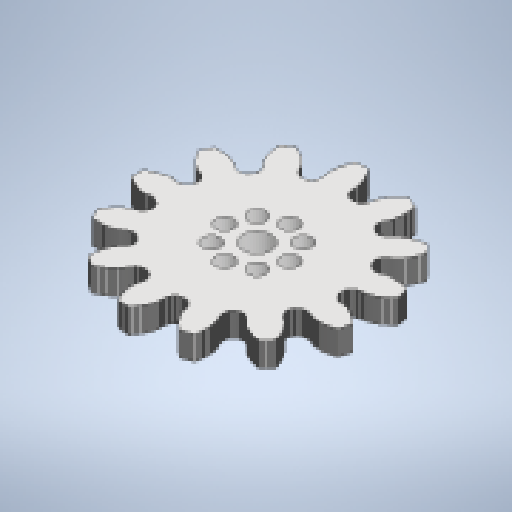
# Autodesk Inventor part: gia1
Saved by Autodesk Inventor 2024 (Build 280153000, 153)
## iProperties
Created: 2024-07-09
Part Number: gia1
Material: 一般
Document SubType Name: Modeling
Designer: right
Density: 1 g/cm^3
Appearance: 既定
Author: right
Autodesk Inventor part; units mm, degrees
(part 1 of 2)
ref_plane "YZ Plane" through (0, 0, 0) normal (1, 0, 0) x (0, 1, 0)
ref_plane "XZ Plane" through (0, 0, 0) normal (0, 1, 0) x (-1, 0, 0)
ref_plane "作業平面1" through (0, 3, 0) normal (0, 1, 0) x (1, 0, 0)
sketch "スケッチ5" plane through (0, 3, 0) normal (0, 1, 0) x (1, 0, 0)
  line L0 (-15.6, 0) -> (15.6, 0)
  line L1 (0, -15.6) -> (0, 15.6)
  line L2 (10.5, 0) -> (10.5, 0.0208)
  line L3 (10.5, 0.0208) -> (10.4999, 0.0416)
  line L4 (10.4999, 0.0416) -> (10.4998, 0.0624)
  line L5 (10.4998, 0.0624) -> (10.4997, 0.0832)
  line L6 (10.4997, 0.0832) -> (10.4995, 0.104)
  line L7 (10.4995, 0.104) -> (10.5112, 0.2583)
  line L8 (10.5112, 0.2583) -> (10.5367, 0.3785)
  line L9 (10.5367, 0.3785) -> (10.5723, 0.481)
  line L10 (10.5723, 0.481) -> (10.6163, 0.5759)
  line L11 (10.6163, 0.5759) -> (10.668, 0.6619)
  line L12 (10.668, 0.6619) -> (10.7267, 0.7429)
  line L13 (10.7267, 0.7429) -> (10.7921, 0.8168)
  line L14 (10.7921, 0.8168) -> (10.8639, 0.8855)
  line L15 (10.8639, 0.8855) -> (10.9417, 0.9492)
  line L16 (10.9417, 0.9492) -> (11.0257, 1.0054)
  line L17 (11.0257, 1.0054) -> (11.1152, 1.0597)
  line L18 (11.1152, 1.0597) -> (11.2106, 1.1065)
  line L19 (11.2106, 1.1065) -> (11.3115, 1.1473)
  line L20 (11.3115, 1.1473) -> (11.4177, 1.1857)
  line L21 (11.4177, 1.1857) -> (11.5292, 1.2172)
  line L22 (11.5292, 1.2172) -> (11.6463, 1.2415)
  line L23 (11.6463, 1.2415) -> (11.7682, 1.263)
  line L24 (11.7682, 1.263) -> (11.895, 1.2797)
  line L25 (11.895, 1.2797) -> (12.027, 1.2893)
  line L26 (12.027, 1.2893) -> (12.1638, 1.2939)
  line L27 (12.1638, 1.2939) -> (12.2934, 1.3227)
  line L28 (12.2934, 1.3227) -> (12.4219, 1.3615)
  line L29 (12.4219, 1.3615) -> (12.5495, 1.4074)
  line L30 (12.5495, 1.4074) -> (12.6764, 1.4593)
  line L31 (12.6764, 1.4593) -> (12.8025, 1.5165)
  line L32 (12.8025, 1.5165) -> (12.928, 1.5786)
  line L33 (12.928, 1.5786) -> (13.0526, 1.6452)
  line L34 (13.0526, 1.6452) -> (13.1766, 1.7162)
  line L35 (13.1766, 1.7162) -> (13.2997, 1.7913)
  line L36 (13.2997, 1.7913) -> (13.422, 1.8703)
  line L37 (13.422, 1.8703) -> (13.5435, 1.9531)
  line L38 (13.5435, 1.9531) -> (13.6642, 2.0397)
  line L39 (13.6642, 2.0397) -> (13.7839, 2.1299)
  line L40 (13.7839, 2.1299) -> (13.9027, 2.2236)
  line L41 (13.9027, 2.2236) -> (14.0206, 2.3209)
  line L42 (14.0206, 2.3209) -> (14.1374, 2.4215)
  line L43 (14.1374, 2.4215) -> (14.2532, 2.5254)
  line L44 (14.2532, 2.5254) -> (14.3679, 2.6326)
  line L45 (14.3679, 2.6326) -> (14.4816, 2.7431)
  line L46 (14.4816, 2.7431) -> (14.594, 2.8567)
  line L47 (14.594, 2.8567) -> (14.5657, 2.9978)
  line L48 (14.5657, 2.9978) -> (14.536, 3.1385)
  line L49 (14.536, 3.1385) -> (14.505, 3.2789)
  line L50 (14.505, 3.2789) -> (14.4726, 3.4191)
  line L51 (14.4726, 3.4191) -> (14.4389, 3.5589)
  line L52 (14.4389, 3.5589) -> (0, 0) construction
  line L53 (0, 0) -> (1.3798, 0.3401) construction
  circle A0 centre (0, 0) radius 13 construction
  line L54 (9.2973, 4.8796) -> (9.3069, 4.8612)
  line L55 (9.3069, 4.8612) -> (9.3165, 4.8427)
  line L56 (9.3165, 4.8427) -> (9.3261, 4.8243)
  line L57 (9.3261, 4.8243) -> (9.3356, 4.8058)
  line L58 (9.3356, 4.8058) -> (9.3451, 4.7873)
  line L59 (9.3451, 4.7873) -> (9.4272, 4.656)
  line L60 (9.4272, 4.656) -> (9.5057, 4.5616)
  line L61 (9.5057, 4.5616) -> (9.5849, 4.4873)
  line L62 (9.5849, 4.4873) -> (9.6679, 4.4237)
  line L63 (9.6679, 4.4237) -> (9.7536, 4.3716)
  line L64 (9.7536, 4.3716) -> (9.8432, 4.3272)
  line L65 (9.8432, 4.3272) -> (9.9355, 4.2921)
  line L66 (9.9355, 4.2921) -> (10.031, 4.2646)
  line L67 (10.031, 4.2646) -> (10.1296, 4.2444)
  line L68 (10.1296, 4.2444) -> (10.23, 4.2337)
  line L69 (10.23, 4.2337) -> (10.3345, 4.2271)
  line L70 (10.3345, 4.2271) -> (10.4407, 4.23)
  line L71 (10.4407, 4.23) -> (10.5491, 4.2408)
  line L72 (10.5491, 4.2408) -> (10.6609, 4.2561)
  line L73 (10.6609, 4.2561) -> (10.7743, 4.2801)
  line L74 (10.7743, 4.2801) -> (10.8892, 4.313)
  line L75 (10.8892, 4.313) -> (11.0071, 4.3506)
  line L76 (11.0071, 4.3506) -> (11.1272, 4.3948)
  line L77 (11.1272, 4.3948) -> (11.2485, 4.4476)
  line L78 (11.2485, 4.4476) -> (11.3718, 4.5071)
  line L79 (11.3718, 4.5071) -> (11.4999, 4.5418)
  line L80 (11.4999, 4.5418) -> (11.6317, 4.5672)
  line L81 (11.6317, 4.5672) -> (11.7661, 4.5858)
  line L82 (11.7661, 4.5858) -> (11.9026, 4.5989)
  line L83 (11.9026, 4.5989) -> (12.0409, 4.6068)
  line L84 (12.0409, 4.6068) -> (12.1808, 4.6101)
  line L85 (12.1808, 4.6101) -> (12.3221, 4.6091)
  line L86 (12.3221, 4.6091) -> (12.4648, 4.6038)
  line L87 (12.4648, 4.6038) -> (12.6087, 4.5946)
  line L88 (12.6087, 4.5946) -> (12.7538, 4.5815)
  line L89 (12.7538, 4.5815) -> (12.8999, 4.5646)
  line L90 (12.8999, 4.5646) -> (13.0469, 4.544)
  line L91 (13.0469, 4.544) -> (13.1949, 4.5198)
  line L92 (13.1949, 4.5198) -> (13.3436, 4.492)
  line L93 (13.3436, 4.492) -> (13.4932, 4.4607)
  line L94 (13.4932, 4.4607) -> (13.6434, 4.4259)
  line L95 (13.6434, 4.4259) -> (13.7942, 4.3877)
  line L96 (13.7942, 4.3877) -> (13.9456, 4.346)
  line L97 (13.9456, 4.346) -> (14.0976, 4.301)
  line L98 (14.0976, 4.301) -> (14.25, 4.2527)
  line L99 (14.25, 4.2527) -> (14.2904, 4.1147)
  line L100 (14.2904, 4.1147) -> (14.3296, 3.9762)
  line L101 (14.3296, 3.9762) -> (14.3673, 3.8375)
  line L102 (14.3673, 3.8375) -> (14.4038, 3.6983)
  line L103 (14.4038, 3.6983) -> (14.4389, 3.5589)
  line L104 (11.0845, 8.0234) -> (11.1511, 8.1561)
  line L105 (9.583, 10.134) -> (9.7277, 10.1785)
  line L106 (9.8746, 10.2203) -> (10.0238, 10.2593)
  line L107 (10.0238, 10.2593) -> (10.1751, 10.2956)
  line L108 (10.1751, 10.2956) -> (10.3285, 10.3291)
  line L109 (9.7277, 10.1785) -> (9.8746, 10.2203)
  line L110 (10.3285, 10.3291) -> (10.484, 10.3598)
  line L111 (10.484, 10.3598) -> (10.6414, 10.3878)
  line L112 (9.4408, 10.0867) -> (9.583, 10.134)
  line L113 (9.301, 10.0366) -> (9.4408, 10.0867)
  line L114 (9.1638, 9.9837) -> (9.301, 10.0366)
  line L115 (8.402, 9.6035) -> (8.5208, 9.6748)
  line L116 (8.5208, 9.6748) -> (8.6431, 9.7428)
  line L117 (8.6431, 9.7428) -> (8.7688, 9.8075)
  line L118 (8.7688, 9.8075) -> (8.8975, 9.8692)
  line L119 (8.8975, 9.8692) -> (9.0293, 9.9279)
  line L120 (9.0293, 9.9279) -> (9.1638, 9.9837)
  line L121 (9.8332, 6.5873) -> (9.9378, 6.661)
  line L122 (9.9378, 6.661) -> (10.0502, 6.7308)
  line L123 (10.0502, 6.7308) -> (10.1692, 6.7985)
  line L124 (10.1692, 6.7985) -> (10.2706, 6.8842)
  line L125 (10.2706, 6.8842) -> (10.3663, 6.9783)
  line L126 (10.3663, 6.9783) -> (10.458, 7.0783)
  line L127 (10.458, 7.0783) -> (10.5462, 7.1832)
  line L128 (10.5462, 7.1832) -> (10.6313, 7.2925)
  line L129 (10.6313, 7.2925) -> (10.7135, 7.4057)
  line L130 (10.7135, 7.4057) -> (10.793, 7.5227)
  line L131 (10.793, 7.5227) -> (10.8697, 7.6431)
  line L132 (9.643, 6.4357) -> (9.7353, 6.5116)
  line L133 (9.7353, 6.5116) -> (9.8332, 6.5873)
  line L134 (9.5588, 6.3559) -> (9.643, 6.4357)
  line L135 (7.8103, 9.0624) -> (7.8932, 9.1656)
  line L136 (7.8932, 9.1656) -> (7.9747, 9.2756)
  line L137 (7.9747, 9.2756) -> (8.072, 9.3659)
  line L138 (8.072, 9.3659) -> (8.1769, 9.4496)
  line L139 (8.1769, 9.4496) -> (8.2872, 9.5285)
  line L140 (8.2872, 9.5285) -> (8.402, 9.6035)
  line L141 (10.8697, 7.6431) -> (10.9439, 7.7667)
  line L142 (10.9439, 7.7667) -> (11.0155, 7.8936)
  line L143 (11.0155, 7.8936) -> (11.0845, 8.0234)
  line L144 (11.1511, 8.1561) -> (11.2152, 8.2916)
  line L145 (11.2152, 8.2916) -> (11.2769, 8.4299)
  line L146 (11.2769, 8.4299) -> (11.336, 8.5707)
  line L147 (11.447, 8.8599) -> (11.4987, 9.0082)
  line L148 (9.4827, 6.2726) -> (9.5588, 6.3559)
  line L149 (7.279, 8.5975) -> (7.3699, 8.6575)
  line L150 (7.3699, 8.6575) -> (7.4618, 8.723)
  line L151 (7.4618, 8.723) -> (7.5511, 8.7969)
  line L152 (7.5511, 8.7969) -> (7.6376, 8.8795)
  line L153 (7.6376, 8.8795) -> (7.7245, 8.9675)
  line L154 (7.7245, 8.9675) -> (7.8103, 9.0624)
  line L155 (9.3496, 6.1039) -> (9.4122, 6.1896)
  line L156 (9.2473, 5.9254) -> (9.2956, 6.0141)
  line L157 (6.7048, 8.4059) -> (6.8028, 8.4177)
  line L158 (6.8028, 8.4177) -> (6.9001, 8.4378)
  line L159 (6.9001, 8.4378) -> (6.9968, 8.4656)
  line L160 (6.9968, 8.4656) -> (7.0907, 8.5029)
  line L161 (7.0907, 8.5029) -> (7.1863, 8.5456)
  line L162 (7.1863, 8.5456) -> (7.279, 8.5975)
  line L163 (5.9818, 8.6295) -> (5.9989, 8.6176)
  line L164 (5.9647, 8.6413) -> (5.9818, 8.6295)
  line L165 (6.0159, 8.6057) -> (6.0329, 8.5938)
  line L166 (5.9989, 8.6176) -> (6.0159, 8.6057)
  line L167 (6.0329, 8.5938) -> (6.0499, 8.5819)
  line L168 (6.6048, 8.4036) -> (6.7048, 8.4059)
  line L169 (6.5047, 8.4099) -> (6.6048, 8.4036)
  line L170 (6.4016, 8.4276) -> (6.5047, 8.4099)
  line L171 (6.297, 8.4566) -> (6.4016, 8.4276)
  line L172 (6.1836, 8.5038) -> (6.297, 8.4566)
  line L173 (6.0499, 8.5819) -> (6.1836, 8.5038)
  line L174 (9.2973, 4.8796) -> (9.2876, 4.898)
  line L175 (9.2485, 4.9714) -> (9.1871, 5.1135)
  line L176 (9.1871, 5.1135) -> (9.1539, 5.2318)
  line L177 (9.1539, 5.2318) -> (9.1378, 5.3391)
  line L178 (9.1378, 5.3391) -> (9.1326, 5.4436)
  line L179 (9.1326, 5.4436) -> (9.1384, 5.5437)
  line L180 (9.1384, 5.5437) -> (9.1528, 5.6427)
  line L181 (9.1528, 5.6427) -> (9.1763, 5.7386)
  line L182 (9.1763, 5.7386) -> (9.208, 5.8328)
  line L183 (9.208, 5.8328) -> (9.2473, 5.9254)
  line L184 (9.2956, 6.0141) -> (9.3496, 6.1039)
  line L185 (9.2583, 4.9531) -> (9.2485, 4.9714)
  line L186 (9.2681, 4.9347) -> (9.2583, 4.9531)
  line L187 (9.2876, 4.898) -> (9.2779, 4.9164)
  line L188 (9.2779, 4.9164) -> (9.2681, 4.9347)
  line L189 (9.4122, 6.1896) -> (9.4827, 6.2726)
  line L190 (11.3927, 8.7141) -> (11.447, 8.8599)
  line L191 (11.4987, 9.0082) -> (11.548, 9.1588)
  line L192 (11.548, 9.1588) -> (11.5948, 9.3117)
  line L193 (11.5948, 9.3117) -> (11.5042, 9.4234)
  line L194 (11.5042, 9.4234) -> (11.4125, 9.5342)
  line L195 (11.4125, 9.5342) -> (11.3198, 9.6442)
  line L196 (11.3198, 9.6442) -> (11.226, 9.7532)
  line L197 (11.226, 9.7532) -> (11.1311, 9.8613)
  line L198 (10.6414, 10.3878) -> (10.7414, 10.2844)
  line L199 (10.7414, 10.2844) -> (10.8403, 10.1801)
  line L200 (10.8403, 10.1801) -> (10.9383, 10.0748)
  line L201 (10.9383, 10.0748) -> (11.0352, 9.9685)
  line L202 (11.0352, 9.9685) -> (11.1311, 9.8613)
  line L203 (11.336, 8.5707) -> (11.3927, 8.7141)
  line L204 (6.0862, 12.2556) -> (6.0835, 12.4041)
  line L205 (3.7758, 13.4267) -> (3.8832, 13.5333)
  line L206 (3.9939, 13.6386) -> (4.1079, 13.7425)
  line L207 (4.1079, 13.7425) -> (4.225, 13.8449)
  line L208 (4.225, 13.8449) -> (4.3453, 13.9459)
  line L209 (3.8832, 13.5333) -> (3.9939, 13.6386)
  line L210 (4.3453, 13.9459) -> (4.4687, 14.0453)
  line L211 (4.4687, 14.0453) -> (4.595, 14.1433)
  line L212 (3.6719, 13.3187) -> (3.7758, 13.4267)
  line L213 (3.5714, 13.2094) -> (3.6719, 13.3187)
  line L214 (3.4745, 13.0987) -> (3.5714, 13.2094)
  line L215 (2.9767, 12.4081) -> (3.0487, 12.5264)
  line L216 (3.0487, 12.5264) -> (3.1254, 12.6434)
  line L217 (3.1254, 12.6434) -> (3.2066, 12.7592)
  line L218 (3.2066, 12.7592) -> (3.2919, 12.8736)
  line L219 (3.2919, 12.8736) -> (3.3813, 12.9868)
  line L220 (3.3813, 12.9868) -> (3.4745, 13.0987)
  line L221 (5.6456, 10.4025) -> (5.704, 10.5164)
  line L222 (5.704, 10.5164) -> (5.7711, 10.6304)
  line L223 (5.7711, 10.6304) -> (5.845, 10.7456)
  line L224 (5.845, 10.7456) -> (5.8949, 10.8686)
  line L225 (5.8949, 10.8686) -> (5.9359, 10.9964)
  line L226 (5.9359, 10.9964) -> (5.9707, 11.1276)
  line L227 (5.9707, 11.1276) -> (6, 11.2615)
  line L228 (6, 11.2615) -> (6.0246, 11.3978)
  line L229 (6.0246, 11.3978) -> (6.0447, 11.5363)
  line L230 (6.0447, 11.5363) -> (6.0607, 11.6767)
  line L231 (6.0607, 11.6767) -> (6.0727, 11.819)
  line L232 (5.5476, 10.1798) -> (5.5941, 10.2899)
  line L233 (5.5941, 10.2899) -> (5.6456, 10.4025)
  line L234 (5.5101, 10.0701) -> (5.5476, 10.1798)
  line L235 (2.7042, 11.654) -> (2.7296, 11.7839)
  line L236 (2.7296, 11.7839) -> (2.7506, 11.9191)
  line L237 (2.7506, 11.9191) -> (2.7948, 12.0443)
  line L238 (2.7948, 12.0443) -> (2.8489, 12.1672)
  line L239 (2.8489, 12.1672) -> (2.9098, 12.2884)
  line L240 (2.9098, 12.2884) -> (2.9767, 12.4081)
  line L241 (6.0727, 11.819) -> (6.0809, 11.963)
  line L242 (6.0809, 11.963) -> (6.0854, 12.1085)
  line L243 (6.0854, 12.1085) -> (6.0862, 12.2556)
  line L244 (6.0835, 12.4041) -> (6.0773, 12.5539)
  line L245 (6.0773, 12.5539) -> (6.0676, 12.7049)
  line L246 (6.0676, 12.7049) -> (6.0546, 12.8571)
  line L247 (6.0184, 13.1648) -> (5.9953, 13.3201)
  line L248 (5.4815, 9.961) -> (5.5101, 10.0701)
  line L249 (2.4497, 10.9955) -> (2.5024, 11.0908)
  line L250 (2.5024, 11.0908) -> (2.5533, 11.1915)
  line L251 (2.5533, 11.1915) -> (2.598, 11.2985)
  line L252 (2.598, 11.2985) -> (2.6362, 11.4117)
  line L253 (2.6362, 11.4117) -> (2.6723, 11.5301)
  line L254 (2.6723, 11.5301) -> (2.7042, 11.654)
  line L255 (5.442, 9.7497) -> (5.4577, 9.8547)
  line L256 (5.4344, 9.5441) -> (5.4359, 9.6451)
  line L257 (2.0304, 10.5589) -> (2.1117, 10.615)
  line L258 (2.1117, 10.615) -> (2.1885, 10.6779)
  line L259 (2.1885, 10.6779) -> (2.2612, 10.7475)
  line L260 (2.2612, 10.7475) -> (2.3271, 10.8242)
  line L261 (2.3271, 10.8242) -> (2.3918, 10.9064)
  line L262 (2.3918, 10.9064) -> (2.4497, 10.9955)
  line L263 (1.2863, 10.4209) -> (1.3069, 10.4183)
  line L264 (1.2656, 10.4234) -> (1.2863, 10.4209)
  line L265 (1.3275, 10.4157) -> (1.3482, 10.4131)
  line L266 (1.3069, 10.4183) -> (1.3275, 10.4157)
  line L267 (1.3482, 10.4131) -> (1.3688, 10.4104)
  line L268 (1.943, 10.5104) -> (2.0304, 10.5589)
  line L269 (1.8514, 10.4695) -> (1.943, 10.5104)
  line L270 (1.7519, 10.4373) -> (1.8514, 10.4695)
  line L271 (1.6458, 10.4143) -> (1.7519, 10.4373)
  line L272 (1.5234, 10.4034) -> (1.6458, 10.4143)
  line L273 (1.3688, 10.4104) -> (1.5234, 10.4034)
  line L274 (5.9647, 8.6413) -> (5.9476, 8.6531)
  line L275 (5.8788, 8.7) -> (5.7584, 8.7973)
  line L276 (5.7584, 8.7973) -> (5.6741, 8.8865)
  line L277 (5.6741, 8.8865) -> (5.6099, 8.9741)
  line L278 (5.6099, 8.9741) -> (5.5568, 9.0642)
  line L279 (5.5568, 9.0642) -> (5.5154, 9.1556)
  line L280 (5.5154, 9.1556) -> (5.4821, 9.2499)
  line L281 (5.4821, 9.2499) -> (5.4584, 9.3457)
  line L282 (5.4584, 9.3457) -> (5.4426, 9.4438)
  line L283 (5.4426, 9.4438) -> (5.4344, 9.5441)
  line L284 (5.4359, 9.6451) -> (5.442, 9.7497)
  line L285 (5.896, 8.6883) -> (5.8788, 8.7)
  line L286 (5.9132, 8.6766) -> (5.896, 8.6883)
  line L287 (5.9476, 8.6531) -> (5.9304, 8.6649)
  line L288 (5.9304, 8.6649) -> (5.9132, 8.6766)
  line L289 (5.4577, 9.8547) -> (5.4815, 9.961)
  line L290 (6.0381, 13.0104) -> (6.0184, 13.1648)
  line L291 (5.9953, 13.3201) -> (5.9689, 13.4764)
  line L292 (5.9689, 13.4764) -> (5.9393, 13.6335)
  line L293 (5.9393, 13.6335) -> (5.8072, 13.6903)
  line L294 (5.8072, 13.6903) -> (5.6745, 13.7458)
  line L295 (5.6745, 13.7458) -> (5.5413, 13.8)
  line L296 (5.5413, 13.8) -> (5.4076, 13.853)
  line L297 (5.4076, 13.853) -> (5.2733, 13.9046)
  line L298 (4.595, 14.1433) -> (4.7316, 14.0982)
  line L299 (4.7316, 14.0982) -> (4.8677, 14.0518)
  line L300 (4.8677, 14.0518) -> (5.0034, 14.004)
  line L301 (5.0034, 14.004) -> (5.1386, 13.955)
  line L302 (5.1386, 13.955) -> (5.2733, 13.9046)
  line L303 (6.0546, 12.8571) -> (6.0381, 13.0104)
  line L304 (-0.3064, 13.6802) -> (-0.3778, 13.8104)
  line L305 (-2.8963, 13.6435) -> (-2.8508, 13.7878)
  line L306 (-2.8017, 13.9324) -> (-2.7491, 14.0774)
  line L307 (-2.7491, 14.0774) -> (-2.693, 14.2225)
  line L308 (-2.693, 14.2225) -> (-2.6334, 14.3678)
  line L309 (-2.8508, 13.7878) -> (-2.8017, 13.9324)
  line L310 (-2.6334, 14.3678) -> (-2.5704, 14.5132)
  line L311 (-2.5704, 14.5132) -> (-2.504, 14.6587)
  line L312 (-2.9382, 13.4995) -> (-2.8963, 13.6435)
  line L313 (-2.9764, 13.356) -> (-2.9382, 13.4995)
  line L314 (-3.0108, 13.213) -> (-2.9764, 13.356)
  line L315 (-3.1306, 12.3701) -> (-3.1219, 12.5084)
  line L316 (-3.1219, 12.5084) -> (-3.1083, 12.6476)
  line L317 (-3.1083, 12.6476) -> (-3.0902, 12.7878)
  line L318 (-3.0902, 12.7878) -> (-3.0678, 12.9289)
  line L319 (-3.0678, 12.9289) -> (-3.0413, 13.0706)
  line L320 (-3.0413, 13.0706) -> (-3.0108, 13.213)
  line L321 (0.1647, 11.8346) -> (0.1634, 11.9625)
  line L322 (0.1634, 11.9625) -> (0.1698, 12.0947)
  line L323 (0.1698, 12.0947) -> (0.1817, 12.2311)
  line L324 (0.1817, 12.2311) -> (0.1688, 12.3632)
  line L325 (0.1688, 12.3632) -> (0.1457, 12.4954)
  line L326 (0.1457, 12.4954) -> (0.1155, 12.6277)
  line L327 (0.1155, 12.6277) -> (0.0793, 12.7599)
  line L328 (0.0793, 12.7599) -> (0.0377, 12.892)
  line L329 (0.0377, 12.892) -> (-0.0088, 13.024)
  line L330 (-0.0088, 13.024) -> (-0.0599, 13.1558)
  line L331 (-0.0599, 13.1558) -> (-0.1154, 13.2873)
  line L332 (0.1814, 11.5919) -> (0.1714, 11.711)
  line L333 (0.1714, 11.711) -> (0.1647, 11.8346)
  line L334 (0.1992, 11.4773) -> (0.1814, 11.5919)
  line L335 (-3.0215, 11.5758) -> (-3.0594, 11.7026)
  line L336 (-3.0594, 11.7026) -> (-3.1035, 11.8322)
  line L337 (-3.1035, 11.8322) -> (-3.1226, 11.9635)
  line L338 (-3.1226, 11.9635) -> (-3.1318, 12.0975)
  line L339 (-3.1318, 12.0975) -> (-3.1342, 12.2331)
  line L340 (-3.1342, 12.2331) -> (-3.1306, 12.3701)
  line L341 (-0.1154, 13.2873) -> (-0.1751, 13.4186)
  line L342 (-0.1751, 13.4186) -> (-0.2388, 13.5496)
  line L343 (-0.2388, 13.5496) -> (-0.3064, 13.6802)
  line L344 (-0.3778, 13.8104) -> (-0.4529, 13.9401)
  line L345 (-0.4529, 13.9401) -> (-0.5316, 14.0694)
  line L346 (-0.5316, 14.0694) -> (-0.6139, 14.1981)
  line L347 (-0.789, 14.4537) -> (-0.8816, 14.5805)
  line L348 (0.2245, 11.3674) -> (0.1992, 11.4773)
  line L349 (-2.9407, 10.8745) -> (-2.9384, 10.9833)
  line L350 (-2.9384, 10.9833) -> (-2.9401, 11.0962)
  line L351 (-2.9401, 11.0962) -> (-2.9502, 11.2117)
  line L352 (-2.9502, 11.2117) -> (-2.969, 11.3297)
  line L353 (-2.969, 11.3297) -> (-2.9921, 11.4513)
  line L354 (-2.9921, 11.4513) -> (-3.0215, 11.5758)
  line L355 (0.2878, 11.1619) -> (0.2528, 11.2622)
  line L356 (0.3766, 10.9764) -> (0.331, 11.0665)
  line L357 (-3.1091, 10.293) -> (-3.0632, 10.3804)
  line L358 (-3.0632, 10.3804) -> (-3.0244, 10.4719)
  line L359 (-3.0244, 10.4719) -> (-2.9924, 10.5673)
  line L360 (-2.9924, 10.5673) -> (-2.9697, 10.6658)
  line L361 (-2.9697, 10.6658) -> (-2.9506, 10.7687)
  line L362 (-2.9506, 10.7687) -> (-2.9407, 10.8745)
  line L363 (-3.7039, 9.825) -> (-3.6844, 9.8323)
  line L364 (-3.7234, 9.8177) -> (-3.7039, 9.825)
  line L365 (-3.665, 9.8396) -> (-3.6455, 9.8469)
  line L366 (-3.6844, 9.8323) -> (-3.665, 9.8396)
  line L367 (-3.6455, 9.8469) -> (-3.626, 9.8541)
  line L368 (-3.164, 10.2095) -> (-3.1091, 10.293)
  line L369 (-3.2261, 10.1307) -> (-3.164, 10.2095)
  line L370 (-3.2992, 10.0559) -> (-3.2261, 10.1307)
  line L371 (-3.3825, 9.9862) -> (-3.2992, 10.0559)
  line L372 (-3.4858, 9.9197) -> (-3.3825, 9.9862)
  line L373 (-3.626, 9.8541) -> (-3.4858, 9.9197)
  line L374 (1.2656, 10.4234) -> (1.245, 10.4259)
  line L375 (1.1624, 10.4355) -> (1.0105, 10.4657)
  line L376 (1.0105, 10.4657) -> (0.8944, 10.5055)
  line L377 (0.8944, 10.5055) -> (0.7968, 10.5532)
  line L378 (0.7968, 10.5532) -> (0.7079, 10.6083)
  line L379 (0.7079, 10.6083) -> (0.6288, 10.67)
  line L380 (0.6288, 10.67) -> (0.5555, 10.738)
  line L381 (0.5555, 10.738) -> (0.49, 10.8119)
  line L382 (0.49, 10.8119) -> (0.4304, 10.8914)
  line L383 (0.4304, 10.8914) -> (0.3766, 10.9764)
  line L384 (0.331, 11.0665) -> (0.2878, 11.1619)
  line L385 (1.183, 10.4331) -> (1.1624, 10.4355)
  line L386 (1.2037, 10.4308) -> (1.183, 10.4331)
  line L387 (1.245, 10.4259) -> (1.2243, 10.4284)
  line L388 (1.2243, 10.4284) -> (1.2037, 10.4308)
  line L389 (0.2528, 11.2622) -> (0.2245, 11.3674)
  line L390 (-0.6997, 14.3262) -> (-0.789, 14.4537)
  line L391 (-0.8816, 14.5805) -> (-0.9775, 14.7066)
  line L392 (-0.9775, 14.7066) -> (-1.0768, 14.832)
  line L393 (-1.0768, 14.832) -> (-1.2202, 14.8209)
  line L394 (-1.2202, 14.8209) -> (-1.3635, 14.8084)
  line L395 (-1.3635, 14.8084) -> (-1.5066, 14.7945)
  line L396 (-1.5066, 14.7945) -> (-1.6496, 14.7792)
  line L397 (-1.6496, 14.7792) -> (-1.7925, 14.7626)
  line L398 (-2.504, 14.6587) -> (-2.3621, 14.6822)
  line L399 (-2.3621, 14.6822) -> (-2.22, 14.7044)
  line L400 (-2.22, 14.7044) -> (-2.0777, 14.7251)
  line L401 (-2.0777, 14.7251) -> (-1.9352, 14.7446)
  line L402 (-1.9352, 14.7446) -> (-1.7925, 14.7626)
  line L403 (-0.6139, 14.1981) -> (-0.6997, 14.3262)
  line L404 (-6.6288, 11.9708) -> (-6.7525, 12.0529)
  line L405 (-8.905, 10.7347) -> (-8.9318, 10.8836)
  line L406 (-8.9555, 11.0345) -> (-8.9763, 11.1873)
  line L407 (-8.9763, 11.1873) -> (-8.994, 11.3419)
  line L408 (-8.994, 11.3419) -> (-9.0088, 11.4983)
  line L409 (-8.9318, 10.8836) -> (-8.9555, 11.0345)
  line L410 (-9.0088, 11.4983) -> (-9.0206, 11.6563)
  line L411 (-9.0206, 11.6563) -> (-9.0294, 11.8159)
  line L412 (-8.8752, 10.5878) -> (-8.905, 10.7347)
  line L413 (-8.8423, 10.443) -> (-8.8752, 10.5878)
  line L414 (-8.8063, 10.3004) -> (-8.8423, 10.443)
  line L415 (-8.5207, 9.4983) -> (-8.5772, 9.6248)
  line L416 (-8.5772, 9.6248) -> (-8.6299, 9.7544)
  line L417 (-8.6299, 9.7544) -> (-8.679, 9.887)
  line L418 (-8.679, 9.887) -> (-8.7247, 10.0223)
  line L419 (-8.7247, 10.0223) -> (-8.7671, 10.1601)
  line L420 (-8.7671, 10.1601) -> (-8.8063, 10.3004)
  line L421 (-5.354, 10.5555) -> (-5.4146, 10.6682)
  line L422 (-5.4146, 10.6682) -> (-5.4703, 10.7883)
  line L423 (-5.4703, 10.7883) -> (-5.5231, 10.9145)
  line L424 (-5.5231, 10.9145) -> (-5.596, 11.0255)
  line L425 (-5.596, 11.0255) -> (-5.6779, 11.1319)
  line L426 (-5.6779, 11.1319) -> (-5.7661, 11.2349)
  line L427 (-5.7661, 11.2349) -> (-5.8596, 11.3352)
  line L428 (-5.8596, 11.3352) -> (-5.9578, 11.4328)
  line L429 (-5.9578, 11.4328) -> (-6.0603, 11.5281)
  line L430 (-6.0603, 11.5281) -> (-6.1669, 11.621)
  line L431 (-6.1669, 11.621) -> (-6.2771, 11.7117)
  line L432 (-5.2264, 10.3484) -> (-5.2906, 10.4492)
  line L433 (-5.2906, 10.4492) -> (-5.354, 10.5555)
  line L434 (-5.1574, 10.2552) -> (-5.2264, 10.3484)
  line L435 (-8.0549, 8.8457) -> (-8.1474, 8.9404)
  line L436 (-8.1474, 8.9404) -> (-8.2467, 9.0346)
  line L437 (-8.2467, 9.0346) -> (-8.3246, 9.1421)
  line L438 (-8.3246, 9.1421) -> (-8.3951, 9.2563)
  line L439 (-8.3951, 9.2563) -> (-8.4602, 9.3753)
  line L440 (-8.4602, 9.3753) -> (-8.5207, 9.4983)
  line L441 (-6.2771, 11.7117) -> (-6.391, 11.8002)
  line L442 (-6.391, 11.8002) -> (-6.5083, 11.8866)
  line L443 (-6.5083, 11.8866) -> (-6.6288, 11.9708)
  line L444 (-6.7525, 12.0529) -> (-6.8793, 12.1329)
  line L445 (-6.8793, 12.1329) -> (-7.0091, 12.2108)
  line L446 (-7.0091, 12.2108) -> (-7.1418, 12.2865)
  line L447 (-7.4156, 12.4315) -> (-7.5565, 12.5007)
  line L448 (-5.0839, 10.1696) -> (-5.1574, 10.2552)
  line L449 (-7.6575, 8.2622) -> (-7.706, 8.3597)
  line L450 (-7.706, 8.3597) -> (-7.76, 8.4588)
  line L451 (-7.76, 8.4588) -> (-7.8226, 8.5564)
  line L452 (-7.8226, 8.5564) -> (-7.8941, 8.6522)
  line L453 (-7.8941, 8.6522) -> (-7.9711, 8.7491)
  line L454 (-7.9711, 8.7491) -> (-8.0549, 8.8457)
  line L455 (-4.9324, 10.0171) -> (-5.0099, 10.0897)
  line L456 (-4.7676, 9.8941) -> (-4.8498, 9.9527)
  line L457 (-7.5364, 7.6692) -> (-7.5364, 7.7679)
  line L458 (-7.5364, 7.7679) -> (-7.5445, 7.8669)
  line L459 (-7.5445, 7.8669) -> (-7.5605, 7.9662)
  line L460 (-7.5605, 7.9662) -> (-7.5862, 8.064)
  line L461 (-7.5862, 8.064) -> (-7.6171, 8.164)
  line L462 (-7.6171, 8.164) -> (-7.6575, 8.2622)
  line L463 (-7.8456, 6.9783) -> (-7.8317, 6.9939)
  line L464 (-7.8594, 6.9628) -> (-7.8456, 6.9783)
  line L465 (-7.8179, 7.0094) -> (-7.804, 7.0248)
  line L466 (-7.8317, 6.9939) -> (-7.8179, 7.0094)
  line L467 (-7.804, 7.0248) -> (-7.79, 7.0403)
  line L468 (-7.5462, 7.5696) -> (-7.5364, 7.6692)
  line L469 (-7.5645, 7.471) -> (-7.5462, 7.5696)
  line L470 (-7.5945, 7.3708) -> (-7.5645, 7.471)
  line L471 (-7.6359, 7.2704) -> (-7.5945, 7.3708)
  line L472 (-7.6964, 7.1636) -> (-7.6359, 7.2704)
  line L473 (-7.79, 7.0403) -> (-7.6964, 7.1636)
  line L474 (-3.7234, 9.8177) -> (-3.7428, 9.8103)
  line L475 (-3.8204, 9.7803) -> (-3.9689, 9.7365)
  line L476 (-3.9689, 9.7365) -> (-4.0902, 9.7178)
  line L477 (-4.0902, 9.7178) -> (-4.1988, 9.7147)
  line L478 (-4.1988, 9.7147) -> (-4.3031, 9.7222)
  line L479 (-4.3031, 9.7222) -> (-4.4018, 9.74)
  line L480 (-4.4018, 9.74) -> (-4.4983, 9.7662)
  line L481 (-4.4983, 9.7662) -> (-4.5907, 9.8011)
  line L482 (-4.5907, 9.8011) -> (-4.6803, 9.8439)
  line L483 (-4.6803, 9.8439) -> (-4.7676, 9.8941)
  line L484 (-4.8498, 9.9527) -> (-4.9324, 10.0171)
  line L485 (-3.801, 9.7879) -> (-3.8204, 9.7803)
  line L486 (-3.7816, 9.7954) -> (-3.801, 9.7879)
  line L487 (-3.7428, 9.8103) -> (-3.7622, 9.8028)
  line L488 (-3.7622, 9.8028) -> (-3.7816, 9.7954)
  line L489 (-5.0099, 10.0897) -> (-5.0839, 10.1696)
  line L490 (-7.2773, 12.36) -> (-7.4156, 12.4315)
  line L491 (-7.5565, 12.5007) -> (-7.7001, 12.5678)
  line L492 (-7.7001, 12.5678) -> (-7.8462, 12.6326)
  line L493 (-7.8462, 12.6326) -> (-7.968, 12.5562)
  line L494 (-7.968, 12.5562) -> (-8.0891, 12.4785)
  line L495 (-8.0891, 12.4785) -> (-8.2094, 12.3997)
  line L496 (-8.2094, 12.3997) -> (-8.3289, 12.3197)
  line L497 (-8.3289, 12.3197) -> (-8.4477, 12.2386)
  line L498 (-9.0294, 11.8159) -> (-8.9147, 11.9027)
  line L499 (-8.9147, 11.9027) -> (-8.7992, 11.9884)
  line L500 (-8.7992, 11.9884) -> (-8.6828, 12.0729)
  line L501 (-8.6828, 12.0729) -> (-8.5657, 12.1563)
  line L502 (-8.5657, 12.1563) -> (-8.4477, 12.2386)
  line L503 (-7.1418, 12.2865) -> (-7.2773, 12.36)
  line L504 (-11.4326, 7.5191) -> (-11.5804, 7.5343)
  line L505 (-12.8737, 5.3667) -> (-12.9666, 5.4862)
  line L506 (-13.0577, 5.6088) -> (-13.1471, 5.7344)
  line L507 (-13.1471, 5.7344) -> (-13.2347, 5.863)
  line L508 (-13.2347, 5.863) -> (-13.3204, 5.9946)
  line L509 (-12.9666, 5.4862) -> (-13.0577, 5.6088)
  line L510 (-13.3204, 5.9946) -> (-13.4043, 6.1291)
  line L511 (-13.4043, 6.1291) -> (-13.4863, 6.2663)
  line L512 (-12.779, 5.2505) -> (-12.8737, 5.3667)
  line L513 (-12.6826, 5.1376) -> (-12.779, 5.2505)
  line L514 (-12.5844, 5.028) -> (-12.6826, 5.1376)
  line L515 (-11.9588, 4.4506) -> (-12.0676, 4.5363)
  line L516 (-12.0676, 4.5363) -> (-12.1745, 4.6266)
  line L517 (-12.1745, 4.6266) -> (-12.2796, 4.7211)
  line L518 (-12.2796, 4.7211) -> (-12.383, 4.8197)
  line L519 (-12.383, 4.8197) -> (-12.4846, 4.922)
  line L520 (-12.4846, 4.922) -> (-12.5844, 5.028)
  line L521 (-9.6461, 6.8583) -> (-9.7521, 6.93)
  line L522 (-9.7521, 6.93) -> (-9.8573, 7.0104)
  line L523 (-9.8573, 7.0104) -> (-9.9627, 7.0976)
  line L524 (-9.9627, 7.0976) -> (-10.0788, 7.162)
  line L525 (-10.0788, 7.162) -> (-10.2007, 7.2181)
  line L526 (-10.2007, 7.2181) -> (-10.3267, 7.2684)
  line L527 (-10.3267, 7.2684) -> (-10.4561, 7.3137)
  line L528 (-10.4561, 7.3137) -> (-10.5885, 7.3545)
  line L529 (-10.5885, 7.3545) -> (-10.7235, 7.3912)
  line L530 (-10.7235, 7.3912) -> (-10.861, 7.424)
  line L531 (-10.861, 7.424) -> (-11.0008, 7.4531)
  line L532 (-9.4369, 6.7342) -> (-9.5406, 6.7936)
  line L533 (-9.5406, 6.7936) -> (-9.6461, 6.8583)
  line L534 (-9.3325, 6.6838) -> (-9.4369, 6.7342)
  line L535 (-11.2431, 4.0892) -> (-11.369, 4.13)
  line L536 (-11.369, 4.13) -> (-11.5007, 4.1673)
  line L537 (-11.5007, 4.1673) -> (-11.6196, 4.2262)
  line L538 (-11.6196, 4.2262) -> (-11.7351, 4.2947)
  line L539 (-11.7351, 4.2947) -> (-11.848, 4.3698)
  line L540 (-11.848, 4.3698) -> (-11.9588, 4.4506)
  line L541 (-11.0008, 7.4531) -> (-11.1428, 7.4786)
  line L542 (-11.1428, 7.4786) -> (-11.2868, 7.5005)
  line L543 (-11.2868, 7.5005) -> (-11.4326, 7.5191)
  line L544 (-11.5804, 7.5343) -> (-11.7298, 7.5462)
  line L545 (-11.7298, 7.5462) -> (-11.8809, 7.5548)
  line L546 (-11.8809, 7.5548) -> (-12.0336, 7.5602)
  line L547 (-12.3433, 7.5613) -> (-12.5003, 7.5572)
  line L548 (-9.2276, 6.6422) -> (-9.3325, 6.6838)
  line L549 (-10.62, 3.7572) -> (-10.7083, 3.821)
  line L550 (-10.7083, 3.821) -> (-10.8021, 3.8837)
  line L551 (-10.8021, 3.8837) -> (-10.9029, 3.9409)
  line L552 (-10.9029, 3.9409) -> (-11.0107, 3.9925)
  line L553 (-11.0107, 3.9925) -> (-11.1239, 4.0426)
  line L554 (-11.1239, 4.0426) -> (-11.2431, 4.0892)
  line L555 (-9.0226, 6.5775) -> (-9.125, 6.6057)
  line L556 (-8.8195, 6.5452) -> (-8.9196, 6.5589)
  line L557 (-10.2372, 3.2883) -> (-10.283, 3.3758)
  line L558 (-10.283, 3.3758) -> (-10.3363, 3.4597)
  line L559 (-10.3363, 3.4597) -> (-10.3966, 3.5402)
  line L560 (-10.3966, 3.5402) -> (-10.4647, 3.6148)
  line L561 (-10.4647, 3.6148) -> (-10.5386, 3.689)
  line L562 (-10.5386, 3.689) -> (-10.62, 3.7572)
  line L563 (-10.1899, 2.533) -> (-10.1849, 2.5532)
  line L564 (-10.1949, 2.5128) -> (-10.1899, 2.533)
  line L565 (-10.1798, 2.5733) -> (-10.1747, 2.5935)
  line L566 (-10.1849, 2.5532) -> (-10.1798, 2.5733)
  line L567 (-10.1747, 2.5935) -> (-10.1695, 2.6136)
  line L568 (-10.1996, 3.1957) -> (-10.2372, 3.2883)
  line L569 (-10.17, 3.0999) -> (-10.1996, 3.1957)
  line L570 (-10.15, 2.9972) -> (-10.17, 3.0999)
  line L571 (-10.14, 2.8891) -> (-10.15, 2.9972)
  line L572 (-10.1439, 2.7663) -> (-10.14, 2.8891)
  line L573 (-10.1695, 2.6136) -> (-10.1439, 2.7663)
  line L574 (-7.8594, 6.9628) -> (-7.8731, 6.9472)
  line L575 (-7.9279, 6.8846) -> (-8.039, 6.7768)
  line L576 (-8.039, 6.7768) -> (-8.1378, 6.7039)
  line L577 (-8.1378, 6.7039) -> (-8.2325, 6.6507)
  line L578 (-8.2325, 6.6507) -> (-8.3283, 6.6088)
  line L579 (-8.3283, 6.6088) -> (-8.424, 6.5788)
  line L580 (-8.424, 6.5788) -> (-8.5217, 6.5571)
  line L581 (-8.5217, 6.5571) -> (-8.6196, 6.5451)
  line L582 (-8.6196, 6.5451) -> (-8.7189, 6.5413)
  line L583 (-8.7189, 6.5413) -> (-8.8195, 6.5452)
  line L584 (-8.9196, 6.5589) -> (-9.0226, 6.5775)
  line L585 (-7.9143, 6.9003) -> (-7.9279, 6.8846)
  line L586 (-7.9006, 6.916) -> (-7.9143, 6.9003)
  line L587 (-7.8731, 6.9472) -> (-7.8869, 6.9316)
  line L588 (-7.8869, 6.9316) -> (-7.9006, 6.916)
  line L589 (-9.125, 6.6057) -> (-9.2276, 6.6422)
  line L590 (-12.1877, 7.5623) -> (-12.3433, 7.5613)
  line L591 (-12.5003, 7.5572) -> (-12.6586, 7.5498)
  line L592 (-12.6586, 7.5498) -> (-12.8182, 7.5393)
  line L593 (-12.8182, 7.5393) -> (-12.8905, 7.415)
  line L594 (-12.8905, 7.415) -> (-12.9616, 7.29)
  line L595 (-12.9616, 7.29) -> (-13.0315, 7.1643)
  line L596 (-13.0315, 7.1643) -> (-13.1002, 7.0379)
  line L597 (-13.1002, 7.0379) -> (-13.1676, 6.9109)
  line L598 (-13.4863, 6.2663) -> (-13.4251, 6.3964)
  line L599 (-13.4251, 6.3964) -> (-13.3626, 6.526)
  line L600 (-13.3626, 6.526) -> (-13.2988, 6.6549)
  line L601 (-13.2988, 6.6549) -> (-13.2338, 6.7832)
  line L602 (-13.2338, 6.7832) -> (-13.1676, 6.9109)
  line L603 (-12.0336, 7.5602) -> (-12.1877, 7.5623)
  line L604 (-13.6174, 1.3448) -> (-13.7552, 1.2896)
  line L605 (-13.8931, -1.2307) -> (-14.0309, -1.1681)
  line L606 (-14.1686, -1.1019) -> (-14.3061, -1.0322)
  line L607 (-14.3061, -1.0322) -> (-14.4434, -0.959)
  line L608 (-14.4434, -0.959) -> (-14.5805, -0.8823)
  line L609 (-14.0309, -1.1681) -> (-14.1686, -1.1019)
  line L610 (-14.5805, -0.8823) -> (-14.7172, -0.8023)
  line L611 (-14.7172, -0.8023) -> (-14.8536, -0.7189)
  line L612 (-13.7552, -1.2896) -> (-13.8931, -1.2307)
  line L613 (-13.6174, -1.3448) -> (-13.7552, -1.2896)
  line L614 (-13.4796, -1.3962) -> (-13.6174, -1.3448)
  line L615 (-12.6573, -1.6167) -> (-12.7935, -1.5914)
  line L616 (-12.7935, -1.5914) -> (-12.9301, -1.5611)
  line L617 (-12.9301, -1.5611) -> (-13.0671, -1.5263)
  line L618 (-13.0671, -1.5263) -> (-13.2044, -1.487)
  line L619 (-13.2044, -1.487) -> (-13.3419, -1.4436)
  line L620 (-13.3419, -1.4436) -> (-13.4796, -1.3962)
  line L621 (-11.7285, 1.59) -> (-11.8556, 1.6041)
  line L622 (-11.8556, 1.6041) -> (-11.9861, 1.6265)
  line L623 (-11.9861, 1.6265) -> (-12.12, 1.6547)
  line L624 (-12.12, 1.6547) -> (-12.2527, 1.6578)
  line L625 (-12.2527, 1.6578) -> (-12.3867, 1.6508)
  line L626 (-12.3867, 1.6508) -> (-12.5217, 1.6368)
  line L627 (-12.5217, 1.6368) -> (-12.6573, 1.6167)
  line L628 (-12.6573, 1.6167) -> (-12.7935, 1.5914)
  line L629 (-12.7935, 1.5914) -> (-12.9301, 1.5611)
  line L630 (-12.9301, 1.5611) -> (-13.0671, 1.5263)
  line L631 (-13.0671, 1.5263) -> (-13.2044, 1.487)
  line L632 (-11.4855, 1.5773) -> (-11.605, 1.5817)
  line L633 (-11.605, 1.5817) -> (-11.7285, 1.59)
  line L634 (-11.3696, 1.5812) -> (-11.4855, 1.5773)
  line L635 (-11.8556, -1.6041) -> (-11.9861, -1.6265)
  line L636 (-11.9861, -1.6265) -> (-12.12, -1.6547)
  line L637 (-12.12, -1.6547) -> (-12.2527, -1.6578)
  line L638 (-12.2527, -1.6578) -> (-12.3867, -1.6508)
  line L639 (-12.3867, -1.6508) -> (-12.5217, -1.6368)
  line L640 (-12.5217, -1.6368) -> (-12.6573, -1.6167)
  line L641 (-13.2044, 1.487) -> (-13.3419, 1.4436)
  line L642 (-13.3419, 1.4436) -> (-13.4796, 1.3962)
  line L643 (-13.4796, 1.3962) -> (-13.6174, 1.3448)
  line L644 (-13.7552, 1.2896) -> (-13.8931, 1.2307)
  line L645 (-13.8931, 1.2307) -> (-14.0309, 1.1681)
  line L646 (-14.0309, 1.1681) -> (-14.1686, 1.1019)
  line L647 (-14.4434, 0.959) -> (-14.5805, 0.8823)
  line L648 (-11.2574, 1.5931) -> (-11.3696, 1.5812)
  line L649 (-11.1496, -1.6085) -> (-11.2574, -1.5931)
  line L650 (-11.2574, -1.5931) -> (-11.3696, -1.5812)
  line L651 (-11.3696, -1.5812) -> (-11.4855, -1.5773)
  line L652 (-11.4855, -1.5773) -> (-11.605, -1.5817)
  line L653 (-11.605, -1.5817) -> (-11.7285, -1.59)
  line L654 (-11.7285, -1.59) -> (-11.8556, -1.6041)
  line L655 (-11.0458, 1.6311) -> (-11.1496, 1.6085)
  line L656 (-10.8509, 1.6969) -> (-10.946, 1.6625)
  line L657 (-10.5928, -1.8458) -> (-10.674, -1.7896)
  line L658 (-10.674, -1.7896) -> (-10.7601, -1.7401)
  line L659 (-10.7601, -1.7401) -> (-10.8509, -1.6969)
  line L660 (-10.8509, -1.6969) -> (-10.946, -1.6625)
  line L661 (-10.946, -1.6625) -> (-11.0458, -1.6311)
  line L662 (-11.0458, -1.6311) -> (-11.1496, -1.6085)
  line L663 (-10.1998, -2.4926) -> (-10.2048, -2.4724)
  line L664 (-10.1949, -2.5128) -> (-10.1998, -2.4926)
  line L665 (-10.2096, -2.4522) -> (-10.2145, -2.432)
  line L666 (-10.2048, -2.4724) -> (-10.2096, -2.4522)
  line L667 (-10.2145, -2.432) -> (-10.2193, -2.4118)
  line L668 (-10.5164, -1.9104) -> (-10.5928, -1.8458)
  line L669 (-10.4456, -1.9814) -> (-10.5164, -1.9104)
  line L670 (-10.3802, -2.0631) -> (-10.4456, -1.9814)
  line L671 (-10.3211, -2.1541) -> (-10.3802, -2.0631)
  line L672 (-10.2676, -2.2647) -> (-10.3211, -2.1541)
  line L673 (-10.2193, -2.4118) -> (-10.2676, -2.2647)
  line L674 (-10.1949, 2.5128) -> (-10.1998, 2.4926)
  line L675 (-10.2193, 2.4118) -> (-10.2676, 2.2647)
  line L676 (-10.2676, 2.2647) -> (-10.3211, 2.1541)
  line L677 (-10.3211, 2.1541) -> (-10.3802, 2.0631)
  line L678 (-10.3802, 2.0631) -> (-10.4456, 1.9814)
  line L679 (-10.4456, 1.9814) -> (-10.5164, 1.9104)
  line L680 (-10.5164, 1.9104) -> (-10.5928, 1.8458)
  line L681 (-10.5928, 1.8458) -> (-10.674, 1.7896)
  line L682 (-10.674, 1.7896) -> (-10.7601, 1.7401)
  line L683 (-10.7601, 1.7401) -> (-10.8509, 1.6969)
  line L684 (-10.946, 1.6625) -> (-11.0458, 1.6311)
  line L685 (-10.2145, 2.432) -> (-10.2193, 2.4118)
  line L686 (-10.2096, 2.4522) -> (-10.2145, 2.432)
  line L687 (-10.1998, 2.4926) -> (-10.2048, 2.4724)
  line L688 (-10.2048, 2.4724) -> (-10.2096, 2.4522)
  line L689 (-11.1496, 1.6085) -> (-11.2574, 1.5931)
  line L690 (-14.3061, 1.0322) -> (-14.4434, 0.959)
  line L691 (-14.5805, 0.8823) -> (-14.7172, 0.8023)
  line L692 (-14.7172, 0.8023) -> (-14.8536, 0.7189)
  line L693 (-14.8536, 0.7189) -> (-14.8599, 0.5752)
  line L694 (-14.8599, 0.5752) -> (-14.8647, 0.4314)
  line L695 (-14.8647, 0.4314) -> (-14.8682, 0.2876)
  line L696 (-14.8682, 0.2876) -> (-14.8703, 0.1438)
  line L697 (-14.8703, 0.1438) -> (-14.871, 0)
  line L698 (-14.8536, -0.7189) -> (-14.8599, -0.5752)
  line L699 (-14.8599, -0.5752) -> (-14.8647, -0.4314)
  line L700 (-14.8647, -0.4314) -> (-14.8682, -0.2876)
  line L701 (-14.8682, -0.2876) -> (-14.8703, -0.1438)
  line L702 (-14.8703, -0.1438) -> (-14.871, 0)
  line L703 (-14.1686, 1.1019) -> (-14.3061, 1.0322)
  line L704 (-12.6826, -5.1376) -> (-12.779, -5.2505)
  line L705 (-11.7298, -7.5462) -> (-11.8809, -7.5548)
  line L706 (-12.0336, -7.5602) -> (-12.1877, -7.5623)
  line L707 (-12.1877, -7.5623) -> (-12.3433, -7.5613)
  line L708 (-12.3433, -7.5613) -> (-12.5003, -7.5572)
  line L709 (-11.8809, -7.5548) -> (-12.0336, -7.5602)
  line L710 (-12.5003, -7.5572) -> (-12.6586, -7.5498)
  line L711 (-12.6586, -7.5498) -> (-12.8182, -7.5393)
  line L712 (-11.5804, -7.5343) -> (-11.7298, -7.5462)
  line L713 (-11.4326, -7.5191) -> (-11.5804, -7.5343)
  line L714 (-11.2868, -7.5005) -> (-11.4326, -7.5191)
  line L715 (-10.4561, -7.3137) -> (-10.5885, -7.3545)
  line L716 (-10.5885, -7.3545) -> (-10.7235, -7.3912)
  line L717 (-10.7235, -7.3912) -> (-10.861, -7.424)
  line L718 (-10.861, -7.424) -> (-11.0008, -7.4531)
  line L719 (-11.0008, -7.4531) -> (-11.1428, -7.4786)
  line L720 (-11.1428, -7.4786) -> (-11.2868, -7.5005)
  line L721 (-11.1239, -4.0426) -> (-11.2431, -4.0892)
  line L722 (-11.2431, -4.0892) -> (-11.369, -4.13)
  line L723 (-11.369, -4.13) -> (-11.5007, -4.1673)
  line L724 (-11.5007, -4.1673) -> (-11.6196, -4.2262)
  line L725 (-11.6196, -4.2262) -> (-11.7351, -4.2947)
  line L726 (-11.7351, -4.2947) -> (-11.848, -4.3698)
  line L727 (-11.848, -4.3698) -> (-11.9588, -4.4506)
  line L728 (-11.9588, -4.4506) -> (-12.0676, -4.5363)
  line L729 (-12.0676, -4.5363) -> (-12.1745, -4.6266)
  line L730 (-12.1745, -4.6266) -> (-12.2796, -4.7211)
  line L731 (-12.2796, -4.7211) -> (-12.383, -4.8197)
  line L732 (-10.9029, -3.9409) -> (-11.0107, -3.9925)
  line L733 (-11.0107, -3.9925) -> (-11.1239, -4.0426)
  line L734 (-10.8021, -3.8837) -> (-10.9029, -3.9409)
  line L735 (-9.7521, -6.93) -> (-9.8573, -7.0104)
  line L736 (-9.8573, -7.0104) -> (-9.9627, -7.0976)
  line L737 (-9.9627, -7.0976) -> (-10.0788, -7.162)
  line L738 (-10.0788, -7.162) -> (-10.2007, -7.2181)
  line L739 (-10.2007, -7.2181) -> (-10.3267, -7.2684)
  line L740 (-10.3267, -7.2684) -> (-10.4561, -7.3137)
  line L741 (-12.383, -4.8197) -> (-12.4846, -4.922)
  line L742 (-12.4846, -4.922) -> (-12.5844, -5.028)
  line L743 (-12.5844, -5.028) -> (-12.6826, -5.1376)
  line L744 (-12.779, -5.2505) -> (-12.8737, -5.3667)
  line L745 (-12.8737, -5.3667) -> (-12.9666, -5.4862)
  line L746 (-12.9666, -5.4862) -> (-13.0577, -5.6088)
  line L747 (-13.2347, -5.863) -> (-13.3204, -5.9946)
  line L748 (-10.7083, -3.821) -> (-10.8021, -3.8837)
  line L749 (-9.125, -6.6057) -> (-9.2276, -6.6422)
  line L750 (-9.2276, -6.6422) -> (-9.3325, -6.6838)
  line L751 (-9.3325, -6.6838) -> (-9.4369, -6.7342)
  line L752 (-9.4369, -6.7342) -> (-9.5406, -6.7936)
  line L753 (-9.5406, -6.7936) -> (-9.6461, -6.8583)
  line L754 (-9.6461, -6.8583) -> (-9.7521, -6.93)
  line L755 (-10.5386, -3.689) -> (-10.62, -3.7572)
  line L756 (-10.3966, -3.5402) -> (-10.4647, -3.6148)
  line L757 (-8.5217, -6.5571) -> (-8.6196, -6.5451)
  line L758 (-8.6196, -6.5451) -> (-8.7189, -6.5413)
  line L759 (-8.7189, -6.5413) -> (-8.8195, -6.5452)
  line L760 (-8.8195, -6.5452) -> (-8.9196, -6.5589)
  line L761 (-8.9196, -6.5589) -> (-9.0226, -6.5775)
  line L762 (-9.0226, -6.5775) -> (-9.125, -6.6057)
  line L763 (-7.8731, -6.9472) -> (-7.8869, -6.9316)
  line L764 (-7.8594, -6.9628) -> (-7.8731, -6.9472)
  line L765 (-7.9006, -6.916) -> (-7.9143, -6.9003)
  line L766 (-7.8869, -6.9316) -> (-7.9006, -6.916)
  line L767 (-7.9143, -6.9003) -> (-7.9279, -6.8846)
  line L768 (-8.424, -6.5788) -> (-8.5217, -6.5571)
  line L769 (-8.3283, -6.6088) -> (-8.424, -6.5788)
  line L770 (-8.2325, -6.6507) -> (-8.3283, -6.6088)
  line L771 (-8.1378, -6.7039) -> (-8.2325, -6.6507)
  line L772 (-8.039, -6.7768) -> (-8.1378, -6.7039)
  line L773 (-7.9279, -6.8846) -> (-8.039, -6.7768)
  line L774 (-10.1949, -2.5128) -> (-10.1899, -2.533)
  line L775 (-10.1695, -2.6136) -> (-10.1439, -2.7663)
  line L776 (-10.1439, -2.7663) -> (-10.14, -2.8891)
  line L777 (-10.14, -2.8891) -> (-10.15, -2.9972)
  line L778 (-10.15, -2.9972) -> (-10.17, -3.0999)
  line L779 (-10.17, -3.0999) -> (-10.1996, -3.1957)
  line L780 (-10.1996, -3.1957) -> (-10.2372, -3.2883)
  line L781 (-10.2372, -3.2883) -> (-10.283, -3.3758)
  line L782 (-10.283, -3.3758) -> (-10.3363, -3.4597)
  line L783 (-10.3363, -3.4597) -> (-10.3966, -3.5402)
  line L784 (-10.4647, -3.6148) -> (-10.5386, -3.689)
  line L785 (-10.1747, -2.5935) -> (-10.1695, -2.6136)
  line L786 (-10.1798, -2.5733) -> (-10.1747, -2.5935)
  line L787 (-10.1899, -2.533) -> (-10.1849, -2.5532)
  line L788 (-10.1849, -2.5532) -> (-10.1798, -2.5733)
  line L789 (-10.62, -3.7572) -> (-10.7083, -3.821)
  line L790 (-13.1471, -5.7344) -> (-13.2347, -5.863)
  line L791 (-13.3204, -5.9946) -> (-13.4043, -6.1291)
  line L792 (-13.4043, -6.1291) -> (-13.4863, -6.2663)
  line L793 (-13.4863, -6.2663) -> (-13.4251, -6.3964)
  line L794 (-13.4251, -6.3964) -> (-13.3626, -6.526)
  line L795 (-13.3626, -6.526) -> (-13.2988, -6.6549)
  line L796 (-13.2988, -6.6549) -> (-13.2338, -6.7832)
  line L797 (-13.2338, -6.7832) -> (-13.1676, -6.9109)
  line L798 (-12.8182, -7.5393) -> (-12.8905, -7.415)
  line L799 (-12.8905, -7.415) -> (-12.9616, -7.29)
  line L800 (-12.9616, -7.29) -> (-13.0315, -7.1643)
  line L801 (-13.0315, -7.1643) -> (-13.1002, -7.0379)
  line L802 (-13.1002, -7.0379) -> (-13.1676, -6.9109)
  line L803 (-13.0577, -5.6088) -> (-13.1471, -5.7344)
  line L804 (-8.8423, -10.443) -> (-8.8752, -10.5878)
  line L805 (-6.8793, -12.1329) -> (-7.0091, -12.2108)
  line L806 (-7.1418, -12.2865) -> (-7.2773, -12.36)
  line L807 (-7.2773, -12.36) -> (-7.4156, -12.4315)
  line L808 (-7.4156, -12.4315) -> (-7.5565, -12.5007)
  line L809 (-7.0091, -12.2108) -> (-7.1418, -12.2865)
  line L810 (-7.5565, -12.5007) -> (-7.7001, -12.5678)
  line L811 (-7.7001, -12.5678) -> (-7.8462, -12.6326)
  line L812 (-6.7525, -12.0529) -> (-6.8793, -12.1329)
  line L813 (-6.6288, -11.9708) -> (-6.7525, -12.0529)
  line L814 (-6.5083, -11.8866) -> (-6.6288, -11.9708)
  line L815 (-5.8596, -11.3352) -> (-5.9578, -11.4328)
  line L816 (-5.9578, -11.4328) -> (-6.0603, -11.5281)
  line L817 (-6.0603, -11.5281) -> (-6.1669, -11.621)
  line L818 (-6.1669, -11.621) -> (-6.2771, -11.7117)
  line L819 (-6.2771, -11.7117) -> (-6.391, -11.8002)
  line L820 (-6.391, -11.8002) -> (-6.5083, -11.8866)
  line L821 (-7.9711, -8.7491) -> (-8.0549, -8.8457)
  line L822 (-8.0549, -8.8457) -> (-8.1474, -8.9404)
  line L823 (-8.1474, -8.9404) -> (-8.2467, -9.0346)
  line L824 (-8.2467, -9.0346) -> (-8.3246, -9.1421)
  line L825 (-8.3246, -9.1421) -> (-8.3951, -9.2563)
  line L826 (-8.3951, -9.2563) -> (-8.4602, -9.3753)
  line L827 (-8.4602, -9.3753) -> (-8.5207, -9.4983)
  line L828 (-8.5207, -9.4983) -> (-8.5772, -9.6248)
  line L829 (-8.5772, -9.6248) -> (-8.6299, -9.7544)
  line L830 (-8.6299, -9.7544) -> (-8.679, -9.887)
  line L831 (-8.679, -9.887) -> (-8.7247, -10.0223)
  line L832 (-7.8226, -8.5564) -> (-7.8941, -8.6522)
  line L833 (-7.8941, -8.6522) -> (-7.9711, -8.7491)
  line L834 (-7.76, -8.4588) -> (-7.8226, -8.5564)
  line L835 (-5.4146, -10.6682) -> (-5.4703, -10.7883)
  line L836 (-5.4703, -10.7883) -> (-5.5231, -10.9145)
  line L837 (-5.5231, -10.9145) -> (-5.596, -11.0255)
  line L838 (-5.596, -11.0255) -> (-5.6779, -11.1319)
  line L839 (-5.6779, -11.1319) -> (-5.7661, -11.2349)
  line L840 (-5.7661, -11.2349) -> (-5.8596, -11.3352)
  line L841 (-8.7247, -10.0223) -> (-8.7671, -10.1601)
  line L842 (-8.7671, -10.1601) -> (-8.8063, -10.3004)
  line L843 (-8.8063, -10.3004) -> (-8.8423, -10.443)
  line L844 (-8.8752, -10.5878) -> (-8.905, -10.7347)
  line L845 (-8.905, -10.7347) -> (-8.9318, -10.8836)
  line L846 (-8.9318, -10.8836) -> (-8.9555, -11.0345)
  line L847 (-8.994, -11.3419) -> (-9.0088, -11.4983)
  line L848 (-7.706, -8.3597) -> (-7.76, -8.4588)
  line L849 (-5.0099, -10.0897) -> (-5.0839, -10.1696)
  line L850 (-5.0839, -10.1696) -> (-5.1574, -10.2552)
  line L851 (-5.1574, -10.2552) -> (-5.2264, -10.3484)
  line L852 (-5.2264, -10.3484) -> (-5.2906, -10.4492)
  line L853 (-5.2906, -10.4492) -> (-5.354, -10.5555)
  line L854 (-5.354, -10.5555) -> (-5.4146, -10.6682)
  line L855 (-7.6171, -8.164) -> (-7.6575, -8.2622)
  line L856 (-7.5605, -7.9662) -> (-7.5862, -8.064)
  line L857 (-4.4983, -9.7662) -> (-4.5907, -9.8011)
  line L858 (-4.5907, -9.8011) -> (-4.6803, -9.8439)
  line L859 (-4.6803, -9.8439) -> (-4.7676, -9.8941)
  line L860 (-4.7676, -9.8941) -> (-4.8498, -9.9527)
  line L861 (-4.8498, -9.9527) -> (-4.9324, -10.0171)
  line L862 (-4.9324, -10.0171) -> (-5.0099, -10.0897)
  line L863 (-3.7428, -9.8103) -> (-3.7622, -9.8028)
  line L864 (-3.7234, -9.8177) -> (-3.7428, -9.8103)
  line L865 (-3.7816, -9.7954) -> (-3.801, -9.7879)
  line L866 (-3.7622, -9.8028) -> (-3.7816, -9.7954)
  line L867 (-3.801, -9.7879) -> (-3.8204, -9.7803)
  line L868 (-4.4018, -9.74) -> (-4.4983, -9.7662)
  line L869 (-4.3031, -9.7222) -> (-4.4018, -9.74)
  line L870 (-4.1988, -9.7147) -> (-4.3031, -9.7222)
  line L871 (-4.0902, -9.7178) -> (-4.1988, -9.7147)
  line L872 (-3.9689, -9.7365) -> (-4.0902, -9.7178)
  line L873 (-3.8204, -9.7803) -> (-3.9689, -9.7365)
  line L874 (-7.8594, -6.9628) -> (-7.8456, -6.9783)
  line L875 (-7.79, -7.0403) -> (-7.6964, -7.1636)
  line L876 (-7.6964, -7.1636) -> (-7.6359, -7.2704)
  line L877 (-7.6359, -7.2704) -> (-7.5945, -7.3708)
  line L878 (-7.5945, -7.3708) -> (-7.5645, -7.471)
  line L879 (-7.5645, -7.471) -> (-7.5462, -7.5696)
  line L880 (-7.5462, -7.5696) -> (-7.5364, -7.6692)
  line L881 (-7.5364, -7.6692) -> (-7.5364, -7.7679)
  line L882 (-7.5364, -7.7679) -> (-7.5445, -7.8669)
  line L883 (-7.5445, -7.8669) -> (-7.5605, -7.9662)
  line L884 (-7.5862, -8.064) -> (-7.6171, -8.164)
  line L885 (-7.804, -7.0248) -> (-7.79, -7.0403)
  line L886 (-7.8179, -7.0094) -> (-7.804, -7.0248)
  line L887 (-7.8456, -6.9783) -> (-7.8317, -6.9939)
  line L888 (-7.8317, -6.9939) -> (-7.8179, -7.0094)
  line L889 (-7.6575, -8.2622) -> (-7.706, -8.3597)
  line L890 (-8.9763, -11.1873) -> (-8.994, -11.3419)
  line L891 (-9.0088, -11.4983) -> (-9.0206, -11.6563)
  line L892 (-9.0206, -11.6563) -> (-9.0294, -11.8159)
  line L893 (-9.0294, -11.8159) -> (-8.9147, -11.9027)
  line L894 (-8.9147, -11.9027) -> (-8.7992, -11.9884)
  line L895 (-8.7992, -11.9884) -> (-8.6828, -12.0729)
  line L896 (-8.6828, -12.0729) -> (-8.5657, -12.1563)
  line L897 (-8.5657, -12.1563) -> (-8.4477, -12.2386)
  line L898 (-7.8462, -12.6326) -> (-7.968, -12.5562)
  line L899 (-7.968, -12.5562) -> (-8.0891, -12.4785)
  line L900 (-8.0891, -12.4785) -> (-8.2094, -12.3997)
  line L901 (-8.2094, -12.3997) -> (-8.3289, -12.3197)
  line L902 (-8.3289, -12.3197) -> (-8.4477, -12.2386)
  line L903 (-8.9555, -11.0345) -> (-8.9763, -11.1873)
  line L904 (-2.9764, -13.356) -> (-2.9382, -13.4995)
  line L905 (-0.4529, -13.9401) -> (-0.5316, -14.0694)
  line L906 (-0.6139, -14.1981) -> (-0.6997, -14.3262)
  line L907 (-0.6997, -14.3262) -> (-0.789, -14.4537)
  line L908 (-0.789, -14.4537) -> (-0.8816, -14.5805)
  line L909 (-0.5316, -14.0694) -> (-0.6139, -14.1981)
  line L910 (-0.8816, -14.5805) -> (-0.9775, -14.7066)
  line L911 (-0.9775, -14.7066) -> (-1.0768, -14.832)
  line L912 (-0.3778, -13.8104) -> (-0.4529, -13.9401)
  line L913 (-0.3064, -13.6802) -> (-0.3778, -13.8104)
  line L914 (-0.2388, -13.5496) -> (-0.3064, -13.6802)
  line L915 (0.0793, -12.7599) -> (0.0377, -12.892)
  line L916 (0.0377, -12.892) -> (-0.0088, -13.024)
  line L917 (-0.0088, -13.024) -> (-0.0599, -13.1558)
  line L918 (-0.0599, -13.1558) -> (-0.1154, -13.2873)
  line L919 (-0.1154, -13.2873) -> (-0.1751, -13.4186)
  line L920 (-0.1751, -13.4186) -> (-0.2388, -13.5496)
  line L921 (-2.9921, -11.4513) -> (-3.0215, -11.5758)
  line L922 (-3.0215, -11.5758) -> (-3.0594, -11.7026)
  line L923 (-3.0594, -11.7026) -> (-3.1035, -11.8322)
  line L924 (-3.1035, -11.8322) -> (-3.1226, -11.9635)
  line L925 (-3.1226, -11.9635) -> (-3.1318, -12.0975)
  line L926 (-3.1318, -12.0975) -> (-3.1342, -12.2331)
  line L927 (-3.1342, -12.2331) -> (-3.1306, -12.3701)
  line L928 (-3.1306, -12.3701) -> (-3.1219, -12.5084)
  line L929 (-3.1219, -12.5084) -> (-3.1083, -12.6476)
  line L930 (-3.1083, -12.6476) -> (-3.0902, -12.7878)
  line L931 (-3.0902, -12.7878) -> (-3.0678, -12.9289)
  line L932 (-2.9502, -11.2117) -> (-2.969, -11.3297)
  line L933 (-2.969, -11.3297) -> (-2.9921, -11.4513)
  line L934 (-2.9401, -11.0962) -> (-2.9502, -11.2117)
  line L935 (0.1634, -11.9625) -> (0.1698, -12.0947)
  line L936 (0.1698, -12.0947) -> (0.1817, -12.2311)
  line L937 (0.1817, -12.2311) -> (0.1688, -12.3632)
  line L938 (0.1688, -12.3632) -> (0.1457, -12.4954)
  line L939 (0.1457, -12.4954) -> (0.1155, -12.6277)
  line L940 (0.1155, -12.6277) -> (0.0793, -12.7599)
  line L941 (-3.0678, -12.9289) -> (-3.0413, -13.0706)
  line L942 (-3.0413, -13.0706) -> (-3.0108, -13.213)
  line L943 (-3.0108, -13.213) -> (-2.9764, -13.356)
  line L944 (-2.9382, -13.4995) -> (-2.8963, -13.6435)
  line L945 (-2.8963, -13.6435) -> (-2.8508, -13.7878)
  line L946 (-2.8508, -13.7878) -> (-2.8017, -13.9324)
  line L947 (-2.693, -14.2225) -> (-2.6334, -14.3678)
  line L948 (-2.9384, -10.9833) -> (-2.9401, -11.0962)
  line L949 (0.2528, -11.2622) -> (0.2245, -11.3674)
  line L950 (0.2245, -11.3674) -> (0.1992, -11.4773)
  line L951 (0.1992, -11.4773) -> (0.1814, -11.5919)